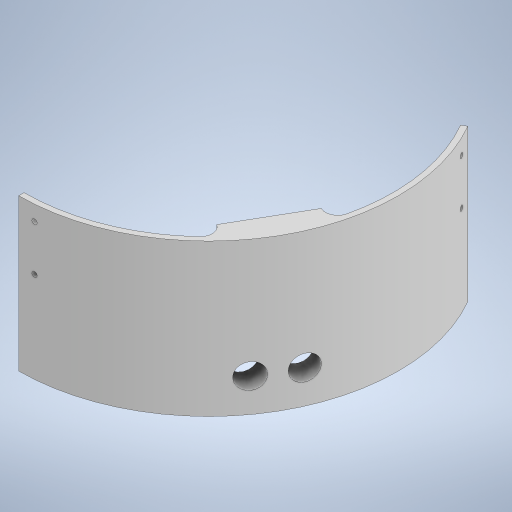
# Autodesk Inventor part: newbody6
Saved by Autodesk Inventor 2023 (Build 270158000, 158)
## iProperties
Created: 2022-11-17
Part Number: newbody6
Material: 一般
Document SubType Name: Modeling
Designer: 野口　裕太
Density: 1 g/cm^3
Appearance: 既定
Author: 野口　裕太
Autodesk Inventor part; units mm, degrees
ref_plane "YZ Plane" through (0, 0, 0) normal (1, 0, 0) x (0, 1, 0)
ref_plane "XZ Plane" through (0, 0, 0) normal (0, 1, 0) x (-1, 0, 0)
ref_plane "XY Plane" through (0, 0, 0) normal (0, 0, 1) x (1, 0, 0)
sketch "スケッチ1" plane through (0, 0, 0) normal (0, 1, 0) x (-1, 0, 0)
  circle A0 centre (0, 0) radius 125
  dimension "d0" = 250
  constraints: 1 centre point, 1 coincident
  measures "d0" diameter of A0
extrude "押し出し1" add sketch "スケッチ1" along normal blind 375
sketch "スケッチ2" plane through (0, 0, 0) normal (0, -1, 0) x (1, 0, 0)
  circle A0 centre (0, 0) radius 125
  constraints: 1 centre point, 1 coincident
extrude "押し出し2" cut sketch "スケッチ2" against normal blind 40
sketch "スケッチ3" plane through (0, 40, 0) normal (0, -1, 0) x (1, 0, 0)
  circle A0 centre (0, 0) radius 125 projected
  point P0 (0, 100)
  point P1 (-86.6025, -50)
  point P2 (86.6025, -50)
  dimension "d5" = 100
  dimension "d8" = 360
  constraints: 4 other
  measures "d5" distance of point (0, 100) A0.centre
hole "穴1" at (0, 40, 100) at (-86.6025, 40, -50) at (86.6025, 40, -50) direction (0, 1, 0) diameter 3.2 depth 8
sketch "スケッチ4" plane through (0, 40, 0) normal (0, -1, 0) x (1, 0, 0)
  circle A0 centre (0, 100) radius 1.6 projected
  point P0 (0, 0)
  point P1 (0, 110)
  point P2 (-95.2628, -55)
  point P3 (95.2628, -55)
  dimension "d17" = 10
  dimension "d20" = 360
  constraints: 4 other
  measures "d17" distance of A0.centre point (0, 110)
hole "穴2" at (0, 40, 110) at (-95.2628, 40, -55) at (95.2628, 40, -55) direction (0, 1, 0) diameter 3.2 depth 8
sketch "スケッチ5" plane through (0, 375, 0) normal (0, 1, 0) x (1, 0, 0)
  circle A0 centre (0, 0) radius 120
  dimension "d29" = 240
  constraints: 1 centre point, 1 coincident
  measures "d29" diameter of A0
extrude "押し出し3" cut sketch "スケッチ5" against normal blind 330
sketch "スケッチ6" plane through (0, 45, 0) normal (0, 1, 0) x (1, 0, 0)
  circle A0 centre (0, 0) radius 120 projected
  line L0 (0, -118) -> (-21.8174, -118)
  line L1 (0, -118) -> (21.8174, -118)
  arc A1 (21.8174, -118) -> (-21.8174, -118) centre (0, 0) ccw
  arc A2 (-21.8174, -118) -> (21.8174, -118) centre (0, 0) ccw
  arc A3 (113.0997, 40.1056) -> (91.2823, 77.8944) centre (0, 0) ccw
  line L2 (102.191, 59) -> (91.2823, 77.8944)
  line L3 (102.191, 59) -> (113.0997, 40.1056)
  arc A4 (-91.2823, 77.8944) -> (-113.0997, 40.1056) centre (0, 0) ccw
  line L4 (-102.191, 59) -> (-113.0997, 40.1056)
  line L5 (-102.191, 59) -> (-91.2823, 77.8944)
  point P0 (-91.2823, 77.8944)
  point P1 (-113.0997, 40.1056)
  point P2 (113.0997, 40.1056)
  point P3 (91.2823, 77.8944)
  dimension "d32" = 118
  dimension "d35" = 360
  constraints: 12 end point, 10 point on circle, 4 centre point, 2 horizontal, 1 coincident, 1 concentric, 22 other
  measures "d32" distance of A0.centre L0.start
extrude "押し出し4" add sketch "スケッチ6" along normal blind 330 contours L3 L2 A0 | A0 L0 L1 | L5 L4 A0
sketch "スケッチ8" plane through (21.8174, 45, 118) normal (0, 0, -1) x (-1, 0, 0)
  line L0 (43.6348, 0) -> (0, 0) projected
  point P0 (21.8174, -45)
  point P1 (11.8174, 60)
  point P2 (31.8174, 60)
  point P3 (11.8174, 90)
  point P4 (31.8174, 90)
  dimension "d52" = 30
  dimension "d90" = 60
  dimension "d91" = 60
  dimension "d92" = 30
  measures "d52" distance of point (11.817, 90) point (11.817, 60)
  measures "d90" distance from line of L0 point (11.817, 60)
  measures "d91" distance from line of L0 point (31.817, 60)
  measures "d92" distance of point (31.817, 60) point (31.817, 90)
hole "穴4" at (10, 105, 118) at (-10, 105, 118) at (10, 135, 118) at (-10, 135, 118) direction (0, 0, 1) diameter 3.2 depth 8
sketch "スケッチ11" plane through (113.0997, 45, -40.1056) normal (-0.8660254, 0, 0.5) x (0.5, 0, 0.8660254)
  line L0 (0, 0) -> (-43.6348, 0) projected
  point P0 (-21.8174, -45)
  point P1 (-31.8174, 60)
  point P2 (-31.8174, 90)
  point P3 (-11.8174, 60)
  point P4 (-11.8174, 90)
  dimension "d65" = 30
  dimension "d95" = 60
  dimension "d96" = 60
  dimension "d98" = 30
  measures "d65" distance of point (-31.817, 60) point (-31.817, 90)
  measures "d95" distance from line of L0 point (-31.817, 60)
  measures "d96" distance from line of L0 point (-11.817, 60)
  measures "d98" distance of point (-11.817, 60) point (-11.817, 90)
hole "穴5" at (97.191, 105, -67.6603) at (97.191, 135, -67.6603) at (107.191, 135, -50.3397) at (107.191, 105, -50.3397) direction (0.8660254, 0, -0.5) diameter 3.2 depth 8
sketch "スケッチ12" plane through (0, 375, 0) normal (0, 1, 0) x (1, 0, 0)
  circle A0 centre (0, 0) radius 121.5
  dimension "d73" = 243
  constraints: 1 centre point, 1 coincident
  measures "d73" diameter of A0
extrude "押し出し6" cut sketch "スケッチ12" against normal blind 330
sketch "スケッチ13" plane through (0, 375, 0) normal (0, 1, 0) x (1, 0, 0)
  circle A0 centre (0, 0) radius 125 projected
  line L0 (0, -125) -> (0, 0)
  line L1 (0, 0) -> (108.2532, 62.5)
  arc A1 (0, -125) -> (108.2532, 62.5) centre (0, 0) ccw
  circle A2 centre (0, 0) radius 125
  dimension "d76" = 125
  dimension "d77" = 120
  constraints: 4 end point, 2 centre point, 2 point on circle, 1 coincident, 1 concentric, 1 vertical, 3 other
  measures "d76" distance of L0.end L1.end
  measures "d77" angle of L0 L1
extrude "押し出し7" cut sketch "スケッチ13" against normal blind 400 contours L1 L0 A0 picked at (69.3351, 45.9431)
sketch "スケッチ14" plane through (0, 45, 0) normal (0, 1, 0) x (1, 0, 0)
  line L0 (0, 0) -> (85.2169, 49.2) projected
  line L1 (0, -111.6) -> (0, -121.5) projected
  circle A0 centre (0, 0) radius 121.5
  constraints: 1 coincident, 1 vertical alignment, 2 other
extrude "押し出し8" cut sketch "スケッチ14" against normal blind 400
sketch "スケッチ15" plane through (0, 40, 0) normal (0, -1, 0) x (1, 0, 0)
  line L0 (0, 0) -> (105.2221, 60.75)
  arc A0 (105.2221, -60.75) -> (0, 121.5) centre (0, 0) ccw projected
  line L1 (0, 0) -> (121.5, 0) construction
  line L2 (102.9357, 59.43) -> (115.531, 37.6143)
  line L3 (102.9357, 59.43) -> (90.3404, 81.2456)
  dimension "d82" = 30
  constraints: 8 end point, 3 point on circle, 2 point on line, 1 equal length, 1 horizontal
  measures "d82" angle of L1 L0
extrude "押し出し9" add sketch "スケッチ15" against normal blind 335
sketch "スケッチ17" plane through (0, 40, 0) normal (0, -1, 0) x (1, 0, 0)
  circle A0 centre (0, 0) radius 125
  constraints: 1 centre point, 1 coincident
extrude "押し出し11" cut sketch "スケッチ17" against normal blind 5
sketch "スケッチ18" plane through (90.3404, 45, 81.2456) normal (-0.8660254, 0, -0.5) x (-0.5, 0, 0.8660254)
  line L0 (-50.3812, 0) -> (0, 0) projected
  circle A0 centre (-38.3406, 22) radius 8.2
  line L1 (-25.1906, 22) -> (-25.1906, 25.3676)
  circle A1 centre (-12.0406, 22) radius 8.2
  point P0 (-25.1906, -45)
  dimension "d99" = 22
  dimension "d100" = 16.4
  dimension "d101" = 13.15
  constraints: 2 centre point, 2 end point, 1 symmetric about line, 1 vertical, 1 other
  measures "d99" distance from line of L0 L1.start
  measures "d100" diameter of A0
  measures "d101" distance of L1.start A0.centre
extrude "押し出し12" cut sketch "スケッチ18" against normal blind 10
sketch "スケッチ19" plane through (0, 375, 0) normal (0, 1, 0) x (1, 0, 0)
  arc A0 (115.531, -37.6143) -> (105.2221, 60.75) centre (0, 0) ccw projected
  line L0 (115.531, -37.6143) -> (90.3404, -81.2456) projected
  line L1 (115.531, -37.6143) -> (90.3404, -81.2456)
  line L2 (90.3404, -81.2456) -> (81.6802, -76.2456)
  line L3 (115.531, -37.6143) -> (106.8708, -32.6143)
  line L4 (106.8708, -32.6143) -> (81.6802, -76.2456)
  dimension "d104" = 10
  constraints: 8 end point, 2 perpendicular, 1 collinear
  measures "d104" distance of L0.end L2.end
extrude "押し出し13" add sketch "スケッチ19" against normal blind 330
sketch "スケッチ20" plane through (106.8708, 45, 32.6143) normal (-0.8660254, 0, -0.5) x (-0.5, 0, 0.8660254)
  circle A0 centre (12.0406, 22) radius 8.2 projected
  circle A1 centre (12.0406, 22) radius 8.2
  circle A2 centre (38.3406, 22) radius 8.2 projected
  circle A3 centre (38.3406, 22) radius 8.2
  point P0 (25.1906, -45)
  constraints: 2 centre point, 2 coincident
extrude "押し出し14" cut sketch "スケッチ20" against normal blind 330
fillet "フィレット1" radius 8 2 edges at (115.531, 210, 37.6143) (90.3404, 210, 81.2456)
sketch "スケッチ21" plane through (0, 375, 0) normal (0, 1, 0) x (1, 0, 0)
  circle A0 centre (0, 0) radius 125
  constraints: 1 centre point, 1 coincident
extrude "押し出し15" cut sketch "スケッチ21" against normal blind 230
sketch "スケッチ22" plane through (106.8708, 45, 32.6143) normal (-0.8660254, 0, -0.5) x (-0.5, 0, 0.8660254)
  line L0 (50.3812, 100) -> (0, 100) projected
  line L1 (25.1906, 85) -> (25.1906, 67.2228)
  point P0 (25.1906, -45)
  point P1 (10.1906, 85)
  point P2 (10.1906, 70)
  point P3 (40.1906, 85)
  point P4 (40.1906, 70)
  dimension "d112" = 15
  dimension "d113" = 15
  dimension "d114" = 15
  dimension "d115" = 15
  constraints: 2 end point, 2 symmetric about line, 1 vertical
  measures "d112" distance from line of L1.start L0
  measures "d113" distance of L1.start point (10.191, 85)
  measures "d114" distance of point (10.191, 85) point (10.191, 70)
  measures "d115" distance from line of L1 point (10.191, 70)
hole "穴6" at (101.7755, 130, 41.4396) at (101.7755, 115, 41.4396) at (86.7755, 130, 67.4204) at (86.7755, 115, 67.4204) direction (0.8660254, 0, 0.5) diameter 2.6 depth 10
sketch "スケッチ23" plane through (0, 45, 0) normal (0, -1, 0) x (1, 0, 0)
  arc A0 (118.386, 27.3315) -> (106.8708, 32.6143) centre (110.591, 25.5319) ccw projected
  line L0 (106.8708, 32.6143) -> (94.2755, 54.4299)
  line L1 (81.6802, 76.2456) -> (106.8708, 32.6143) projected
  line L2 (106.8708, 32.6143) -> (132.0613, 32.6143) construction
  line L3 (94.2755, 54.4299) -> (101.2037, 58.4299)
  line L4 (101.2037, 58.4299) -> (96.2037, 67.0902)
  line L5 (101.2037, 58.4299) -> (111.2037, 58.4299) construction
  line L6 (96.2037, 67.0902) -> (106.2037, 49.7696)
  point P0 (0, 0)
  dimension "d123" = 25.1905
  dimension "d124" = 120
  dimension "d125" = 8
  dimension "d126" = 90
  dimension "d127" = 10
  dimension "d128" = 120
  dimension "d129" = 20
  constraints: 12 end point, 3 coincident, 2 equal length, 2 horizontal, 1 collinear, 1 perpendicular, 1 point on line
  measures "d123" distance of L0.start L0.end
  measures "d124" angle of L2 L0
  measures "d125" distance of L0.end L3.end
  measures "d126" angle of L0 L3
  measures "d127" distance of L4.start L4.end
  measures "d128" angle of L5 L4
  measures "d129" distance of L4.end L6.end
hole "穴7" at (101.2037, 45, 58.4299) at (96.2037, 45, 67.0902) at (106.2037, 45, 49.7696) direction (0, 1, 0) diameter 3.2 depth 10
